# Autodesk Inventor part: esc
Saved by Autodesk Inventor 2021 (Build 250183000, 183)
## iProperties
Created: 2021-01-20
Part Number: esc
Material: Generic
Document SubType Name: Modeling
Designer: User
Density: 1 g/cm^3
Appearance: Default
Author: User
Autodesk Inventor part; units mm, degrees
ref_plane "YZ Plane" through (0, 0, 0) normal (1, 0, 0) x (0, 1, 0)
ref_plane "XZ Plane" through (0, 0, 0) normal (0, 1, 0) x (-1, 0, 0)
ref_plane "XY Plane" through (0, 0, 0) normal (0, 0, 1) x (1, 0, 0)
sketch "Sketch8" plane through (0, 0, 0) normal (0, 1, 0) x (-1, 0, 0)
  line L0 (12.5, 21) -> (-12.5, 21)
  line L1 (-12.5, 21) -> (-12.5, -21)
  line L2 (-12.5, -21) -> (12.5, -21)
  line L3 (12.5, -21) -> (12.5, 21)
  line L4 (12.5, 21) -> (-12.5, -21) construction
  line L5 (-12.5, 21) -> (12.5, -21) construction
  point P0 (0, 0)
  dimension "d63" = 42
  dimension "d64" = 25
  constraints: 12 end point, 2 midpoint, 2 parallel, 1 horizontal, 1 perpendicular
  measures "d63" distance of L0.end L1.end
  measures "d64" distance of L1.end L2.end
extrude "Extrusion8" add sketch "Sketch8" along normal blind 2
body "Solid2"
